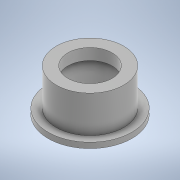
# Autodesk Inventor part: Idle pulley
Saved by Autodesk Inventor 2022 (Build 260153000, 153)
## iProperties
Created: 2022-02-18
Part Number: Idle pulley
Material: Genérico
Document SubType Name: Modeling
Designer: JK
Density: 1 g/cm^3
Appearance: Suave - Gris medio
Mass: 1.63336 g
Surface Area: 17.7666 cm^2
Volume: 1.63336 cm^3
Author: JK
Autodesk Inventor part; units mm, degrees
ref_plane "YZ Plane" through (0, 0, 0) normal (1, 0, 0) x (0, 1, 0)
ref_plane "XZ Plane" through (0, 0, 0) normal (0, 1, 0) x (-1, 0, 0)
ref_plane "XY Plane" through (0, 0, 0) normal (0, 0, 1) x (1, 0, 0)
sketch "Boceto1" plane through (0, 0, 0) normal (0, 1, 0) x (-1, 0, 0)
  circle A0 centre (0, 0) radius 6.05
  circle A1 centre (0, 0) radius 6.85
  dimension "d0" = 12.1
  dimension "d1" = 0.8
  constraints: 2 centre point, 2 coincident
  measures "d0" diameter of A0
  measures "d1" radial gap between concentric circles of A0 A1
extrude "Extrusión1" add sketch "Boceto1" along normal mid plane 6.35
sketch "Boceto2" plane through (0, 3.175, 0) normal (0, 1, 0) x (1, 0, 0)
  circle A0 centre (0, 0) radius 6.05 projected
  circle A1 centre (0, 0) radius 8.5
  dimension "d4" = 17
  constraints: 1 centre point, 1 coincident
  measures "d4" diameter of A1
extrude "Extrusión2" add sketch "Boceto2" along normal blind 1.12
sketch "Boceto3" plane through (0, -3.175, 0) normal (0, -1, 0) x (1, 0, 0)
  circle A0 centre (0, 0) radius 6.05 projected
  circle A1 centre (0, 0) radius 8.5
  circle A2 centre (0, 0) radius 8.5 projected
  constraints: 1 centre point, 1 coincident, 1 concentric
extrude "Extrusión3" add sketch "Boceto3" along normal blind 1.12
sketch "Boceto4" plane through (0, 4.295, 0) normal (0, 1, 0) x (1, 0, 0)
  circle A0 centre (0, 0) radius 6.05 projected
  circle A1 centre (0, 0) radius 4.5
  dimension "d14" = 9
  constraints: 1 centre point, 1 coincident
  measures "d14" diameter of A1
extrude "Extrusión4" add sketch "Boceto4" against normal blind 2.295
sketch "Boceto6" plane through (0, 3.175, 0) normal (0, -1, 0) x (1, 0, 0)
  circle A0 centre (0, 0) radius 6.85 projected
  circle A1 centre (0, 0) radius 8.53
  circle A2 centre (0, 0) radius 7.78
  dimension "d17" = 1.68
  dimension "d18" = 0.75
  constraints: 2 centre point, 2 coincident
  measures "d17" radial gap between concentric circles of A1 A0
  measures "d18" radial gap between concentric circles of A1 A2
fillet "Empalme1" radius 1 1 edges at (-6.05, -4.295, 0)
sketch "Boceto7" plane through (0, 4.295, 0) normal (0, 1, 0) x (1, 0, 0)
  circle A0 centre (0, 0) radius 8.5 projected
  circle A1 centre (0, 0) radius 6.85 projected
  circle A2 centre (0, 0) radius 6.85 projected
extrude "Extrusión6" cut sketch "Boceto7" against normal up to surface (7.47 mm away)
sketch "Boceto5" plane through (0, -4.295, 0) normal (0, -1, 0) x (1, 0, 0)
  circle A0 centre (0, 0) radius 8.5 projected
  circle A1 centre (0, 0) radius 6.85 projected
